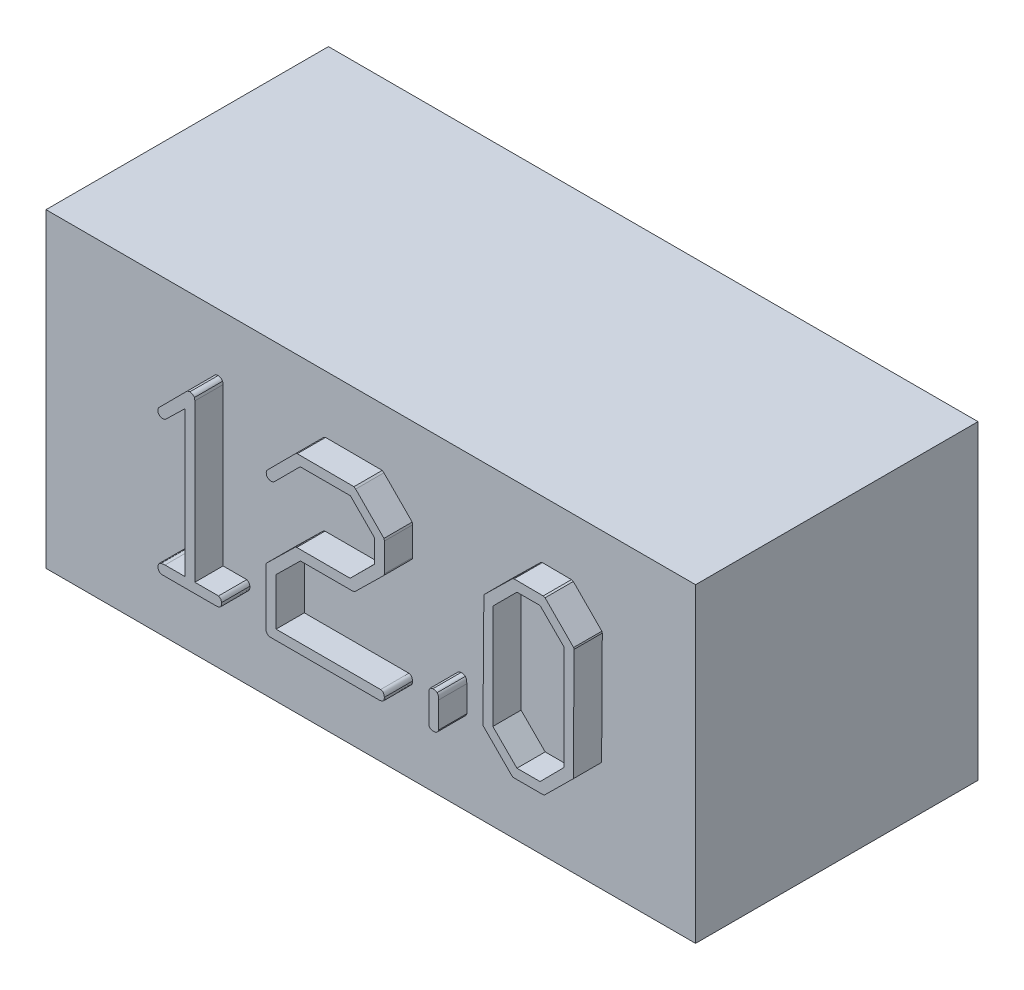
# Autodesk Inventor part: VolteMeter
Saved by Autodesk Inventor 2023 (Build 270158000, 158)
## iProperties
Created: 2022-10-22
Part Number: VolteMeter
Material: Generic
Document SubType Name: Modeling
Designer: Miner
Density: 1 g/cm^3
Appearance: Default
Author: Miner
Autodesk Inventor part; units mm, degrees
ref_plane "YZ Plane" through (0, 0, 0) normal (1, 0, 0) x (0, 1, 0)
ref_plane "XZ Plane" through (0, 0, 0) normal (0, 1, 0) x (-1, 0, 0)
ref_plane "XY Plane" through (0, 0, 0) normal (0, 0, 1) x (1, 0, 0)
sketch "Sketch1" plane through (0, 0, 0) normal (0, 0, 1) x (1, 0, 0)
  line L0 (0, 0) -> (-23, 0)
  line L1 (-23, 0) -> (-23, 11)
  line L2 (-23, 11) -> (0, 11)
  line L3 (0, 11) -> (0, 0)
  line L4 (-17.8694, 8.961) -> (2.181, 8.961) construction
  line L5 (2.181, 8.961) -> (2.181, 1.8992) construction
  line L6 (2.181, 1.8992) -> (-17.8694, 1.8992) construction
  line L7 (-17.8694, 1.8992) -> (-17.8694, 8.961) construction
  line L8 (-16.745, 8.867) -> (-16.7294, 8.7729)
  line L9 (-16.7294, 8.7729) -> (-16.7294, 3.2097)
  line L10 (-16.7294, 3.2097) -> (-15.891, 3.2097)
  spline S0 degree 2 poles (-15.891, 3.2097) (-15.793, 3.1744) (-15.7773, 3.0647) knots 0 0 0 1 1 1
  spline S1 degree 2 poles (-15.7773, 3.0647) (-15.7773, 2.9707) (-15.8518, 2.861) (-15.9693, 2.861) knots 0 0 0 1 2 2 2
  line L11 (-15.9693, 2.861) -> (-17.9204, 2.861)
  spline S2 degree 2 poles (-17.9204, 2.861) (-18.0222, 2.8923) (-18.0379, 3.002) knots 0 0 0 1 1 1
  spline S3 degree 2 poles (-18.0379, 3.002) (-18.0379, 3.1) (-17.9478, 3.2097) (-17.7872, 3.2097) knots 0 0 0 1 2 2 2
  line L12 (-17.7872, 3.2097) -> (-17.078, 3.2097)
  line L13 (-17.078, 3.2097) -> (-17.078, 8.3577)
  line L14 (-17.078, 8.3577) -> (-17.7832, 7.672)
  spline S4 degree 2 poles (-17.7832, 7.672) (-17.8303, 7.6564) (-17.8655, 7.6564) knots 0 0 0 1 1 1
  spline S5 degree 2 poles (-17.8655, 7.6564) (-17.94, 7.6564) (-18.0379, 7.7465) (-18.0379, 7.8366) knots 0 0 0 1 2 2 2
  line L15 (-18.0379, 7.8366) -> (-18.0222, 7.911)
  line L16 (-18.0222, 7.911) -> (-16.9958, 8.9414)
  spline S6 degree 2 poles (-16.9958, 8.9414) (-16.9605, 8.9649) (-16.9017, 8.9649) knots 0 0 0 1 1 1
  spline S7 degree 2 poles (-16.9017, 8.9649) (-16.8861, 8.9649) (-16.7725, 8.914) (-16.745, 8.867) knots 0 0 0 1 2 2 2
  line L17 (-11.0368, 8.914) -> (-10.0339, 7.9032)
  line L18 (-10.0339, 7.9032) -> (-10.0182, 7.8288)
  line L19 (-10.0182, 7.8288) -> (-10.0182, 6.8258)
  line L20 (-10.0182, 6.8258) -> (-10.0339, 6.767)
  line L21 (-10.0339, 6.767) -> (-11.0642, 5.7562)
  line L22 (-11.0642, 5.7562) -> (-11.1387, 5.7327)
  line L23 (-11.1387, 5.7327) -> (-12.9918, 5.7327)
  line L24 (-12.9918, 5.7327) -> (-13.8537, 4.8826)
  line L25 (-13.8537, 4.8826) -> (-13.8537, 3.2097)
  line L26 (-13.8537, 3.2097) -> (-10.1514, 3.2097)
  spline S8 degree 2 poles (-10.1514, 3.2097) (-10.0182, 3.194) (-10.0182, 3.0373) knots 0 0 0 1 1 1
  spline S9 degree 2 poles (-10.0182, 3.0373) (-10.0182, 2.9589) (-10.0848, 2.861) (-10.2023, 2.861) knots 0 0 0 1 2 2 2
  line L27 (-10.2023, 2.861) -> (-14.0927, 2.861)
  spline S10 degree 2 poles (-14.0927, 2.861) (-14.1789, 2.8923) (-14.2024, 2.9668) knots 0 0 0 1 1 1
  line L28 (-14.2024, 2.9668) -> (-14.2024, 3.1352)
  line L29 (-14.2024, 3.1352) -> (-14.2024, 5.055)
  line L30 (-14.2024, 5.055) -> (-13.172, 6.0658)
  line L31 (-13.172, 6.0658) -> (-13.1211, 6.0814)
  line L32 (-13.1211, 6.0814) -> (-11.2327, 6.0814)
  line L33 (-11.2327, 6.0814) -> (-10.3669, 6.9433)
  line L34 (-10.3669, 6.9433) -> (-10.3669, 7.7543)
  line L35 (-10.3669, 7.7543) -> (-11.2209, 8.6162)
  line L36 (-11.2209, 8.6162) -> (-12.9996, 8.6162)
  line L37 (-12.9996, 8.6162) -> (-13.9438, 7.672)
  spline S11 degree 2 poles (-13.9438, 7.672) (-13.9947, 7.6564) (-14.03, 7.6564) knots 0 0 0 1 1 1
  spline S12 degree 2 poles (-14.03, 7.6564) (-14.1044, 7.6564) (-14.2024, 7.7465) (-14.2024, 7.8366) knots 0 0 0 1 2 2 2
  line L38 (-14.2024, 7.8366) -> (-14.1867, 7.911)
  line L39 (-14.1867, 7.911) -> (-13.1681, 8.9336)
  line L40 (-13.1681, 8.9336) -> (-13.1015, 8.9649)
  line L41 (-13.1015, 8.9649) -> (-11.0956, 8.9571)
  line L42 (-11.0956, 8.9571) -> (-11.0368, 8.914)
  spline S13 degree 2 poles (-8.1494, 4.1147) (-8.0985, 4.0716) (-8.0985, 3.9149) knots 0 0 0 1 1 1
  line L43 (-8.0985, 3.9149) -> (-8.0985, 2.9942)
  spline S14 degree 2 poles (-8.0985, 2.9942) (-8.1063, 2.9276) (-8.1886, 2.8767) knots 0 0 0 1 1 1
  spline S15 degree 2 poles (-8.1886, 2.8767) (-8.216, 2.861) (-8.2708, 2.861) knots 0 0 0 1 1 1
  spline S16 degree 2 poles (-8.2708, 2.861) (-8.357, 2.861) (-8.4471, 2.9354) (-8.4471, 3.0451) knots 0 0 0 1 2 2 2
  line L44 (-8.4471, 3.0451) -> (-8.4471, 4.0442)
  spline S17 degree 2 poles (-8.4471, 4.0442) (-8.4158, 4.1617) (-8.2983, 4.1617) knots 0 0 0 1 1 1
  spline S18 degree 2 poles (-8.2983, 4.1617) (-8.1964, 4.1617) (-8.1494, 4.1147) knots 0 0 0 1 1 1
  line L45 (-4.3296, 8.9336) -> (-3.3188, 7.9149)
  line L46 (-3.3188, 7.9149) -> (-3.3031, 7.864)
  line L47 (-3.3031, 7.864) -> (-3.3266, 3.8875)
  line L48 (-3.3266, 3.8875) -> (-4.357, 2.8688)
  line L49 (-4.357, 2.8688) -> (-4.4118, 2.861)
  line L50 (-4.4118, 2.861) -> (-5.4579, 2.861)
  line L51 (-5.4579, 2.861) -> (-5.5088, 2.8923)
  line L52 (-5.5088, 2.8923) -> (-6.5196, 3.911)
  line L53 (-6.5196, 3.911) -> (-6.5274, 3.9972)
  line L54 (-6.5274, 3.9972) -> (-6.4961, 7.9463)
  line L55 (-6.4961, 7.9463) -> (-5.4735, 8.9492)
  line L56 (-5.4735, 8.9492) -> (-5.4265, 8.9649)
  line L57 (-5.4265, 8.9649) -> (-4.3962, 8.9571)
  line L58 (-4.3962, 8.9571) -> (-4.3296, 8.9336)
  line L59 (-3.6518, 7.7543) -> (-4.5059, 8.6084)
  line L60 (-4.5059, 8.6084) -> (-5.3247, 8.6084)
  line L61 (-5.3247, 8.6084) -> (-6.1787, 7.7543)
  line L62 (-6.1787, 7.7543) -> (-6.1787, 4.0638)
  line L63 (-6.1787, 4.0638) -> (-5.3247, 3.2097)
  line L64 (-5.3247, 3.2097) -> (-4.5059, 3.2097)
  line L65 (-4.5059, 3.2097) -> (-3.6518, 4.0716)
  line L66 (-3.6518, 4.0716) -> (-3.6518, 7.7543)
  dimension "d0" = 23
  dimension "d1" = 11
  constraints: 8 end point, 2 parallel, 1 horizontal, 1 perpendicular, 2 other
  measures "d0" distance of L1.end L2.end
  measures "d1" distance of L0.end L1.end
extrude "Extrusion1" add sketch "Sketch1" against normal blind 10 contours L0 L1 L2 L3 | L8 L9 L10 S0 S1 L11 S2 S3 L12 L13 L14 S4 S5 L15 L16 S6 S7 | L17 L18 L19 L20 L21 L22 L23 L24 L25 L26 S8 S9 L27 S10 L28 L29 L30 L31 L32 L33 L34 L35 L36 L37 S11 S12 L38 L39 L40 L41 L42 | S13 L43 S14 S15 S16 L44 S17 S18 | L45 L46 L47 L48 L49 L50 L51 L52 L53 L54 L55 L56 L57 L58 | L66 L65 L64 L63 L62 L61 L60 L59
extrude "Extrusion2" add sketch "Sketch1" along normal blind 1 contours L8 L9 L10 S0 S1 L11 S2 S3 L12 L13 L14 S4 S5 L15 L16 S6 S7 | L17 L18 L19 L20 L21 L22 L23 L24 L25 L26 S8 S9 L27 S10 L28 L29 L30 L31 L32 L33 L34 L35 L36 L37 S11 S12 L38 L39 L40 L41 L42 | S13 L43 S14 S15 S16 L44 S17 S18 | L45 L46 L47 L48 L49 L50 L51 L52 L53 L54 L55 L56 L57 L58
body "Solid1"
